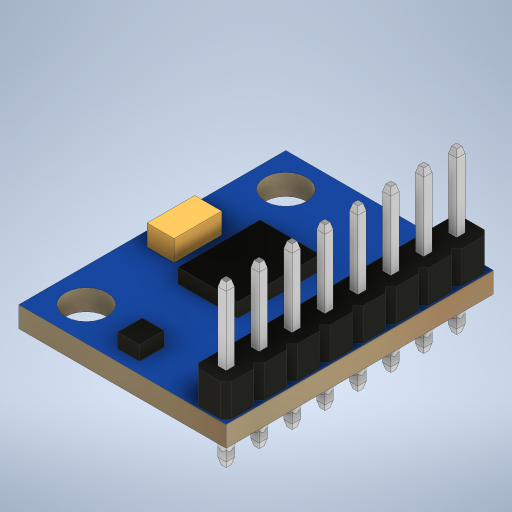
# Autodesk Inventor part: ACCELEROMETER
Saved by Autodesk Inventor 2023 (Build 270158000, 158)
## iProperties
Created: 2023-03-15
Part Number: ACCELEROMETER
Material: Generic
Document SubType Name: Modeling
Designer: Amos Yu
Density: 1 g/cm^3
Appearance: Default
Author: Amos Yu
Autodesk Inventor part; units mm, degrees
ref_plane "YZ Plane" through (0, 0, 0) normal (1, 0, 0) x (0, 1, 0)
ref_plane "XZ Plane" through (0, 0, 0) normal (0, 1, 0) x (-1, 0, 0)
ref_plane "XY Plane" through (0, 0, 0) normal (0, 0, 1) x (1, 0, 0)
sketch "Sketch1" plane through (0, 0, 0) normal (0, 1, 0) x (-1, 0, 0)
  line L0 (0, 0) -> (16, 0)
  line L1 (16, 0) -> (16, -20.6)
  line L2 (16, -20.6) -> (0, -20.6)
  line L3 (0, -20.6) -> (0, 0)
  circle A0 centre (13.4, -2.6) radius 1.6
  circle A1 centre (13.4, -18) radius 1.6
  point P0 (0, -10.3)
  dimension "d0" = 16
  dimension "d1" = 20.6
  dimension "d2" = 3.2
  dimension "d3" = 3.2
  dimension "d6" = 2.6
  dimension "d7" = 2.6
  dimension "d8" = 2.6
  constraints: 8 end point, 2 centre point, 2 parallel, 1 horizontal, 1 midpoint, 1 perpendicular, 1 vertical alignment
  measures "d0" distance of L1.end L2.end
  measures "d1" distance of L0.end L1.end
  measures "d2" diameter of A0
  measures "d3" diameter of A1
  measures "d6" distance from line of L0 A0.centre
  measures "d7" distance from line of L1 A0.centre
  measures "d8" distance from line of L2 A1.centre
extrude "Extrusion1" add sketch "Sketch1" along normal blind 1.6
sketch "Sketch2" plane through (0, 1.6, 0) normal (0, 1, 0) x (1, 0, 0)
  line L0 (-9.2513, 2.7827) -> (-7.5651, 2.7827)
  line L1 (-7.5651, 2.7827) -> (-7.5651, 0.8699)
  line L2 (-7.5651, 0.8699) -> (-9.2513, 0.8699)
  line L3 (-9.2513, 0.8699) -> (-9.2513, 2.7827)
  line L4 (-11.2621, 13.8736) -> (-6.6408, 13.8736)
  line L5 (-6.6408, 13.8736) -> (-6.6408, 7.5359)
  line L6 (-6.6408, 7.5359) -> (-11.2621, 7.5359)
  line L7 (-11.2621, 7.5359) -> (-11.2621, 13.8736)
  line L8 (-14.9036, 12.478) -> (-12.8178, 12.478)
  line L9 (-12.8178, 12.478) -> (-12.8178, 8.8062)
  line L10 (-12.8178, 8.8062) -> (-14.9036, 8.8062)
  line L11 (-14.9036, 8.8062) -> (-14.9036, 12.478)
  line L12 (-16, 20.6) -> (-16, 0) projected
  line L13 (-16, 0) -> (0, 0) projected
  point P0 (-8, 0)
  dimension "d11" = 1.6862
  dimension "d12" = 1.9128
  dimension "d13" = 6.3377
  dimension "d14" = 4.6212
  dimension "d15" = 2.0858
  dimension "d16" = 3.6718
  dimension "d17" = 1.0964
  dimension "d18" = 1.5558
  dimension "d19" = 7.5359
  dimension "d20" = 8.8062
  dimension "d21" = 0.8699
  dimension "d22" = 6.7487
  constraints: 24 end point, 6 parallel, 3 horizontal, 3 perpendicular, 1 midpoint
  measures "d11" distance of L1.end L2.end
  measures "d12" distance of L0.end L1.end
  measures "d13" distance of L4.end L5.end
  measures "d14" distance of L5.end L6.end
  measures "d15" distance of L9.end L10.end
  measures "d16" distance of L8.end L9.end
  measures "d17" distance between parallel lines of L12 L11
  measures "d18" distance between parallel lines of L9 L7
  measures "d19" distance between parallel lines of L13 L6
  measures "d20" distance between parallel lines of L13 L10
  measures "d21" distance from line of point (-8, 0) L2
  measures "d22" distance between parallel lines of L12 L3
extrude "Extrusion2" add sketch "Sketch2" along normal blind 1.1 contours L0 L1 L2 L3 | L4 L5 L6 L7
extrude "Extrusion3" add sketch "Sketch2" along normal blind 1.6 contours L8 L9 L10 L11
sketch "Sketch3" plane through (0, 1.6, 0) normal (0, 1, 0) x (1, 0, 0)
  line L0 (-2.2798, 0.14) -> (-0.5402, 0.14)
  line L1 (-0.5402, 0.14) -> (-0.14, 0.5402)
  line L2 (-0.14, 0.5402) -> (-0.14, 2.2798)
  line L3 (-0.14, 2.2798) -> (-0.5402, 2.68)
  line L4 (-0.5402, 2.68) -> (-2.2798, 2.68)
  line L5 (-2.2798, 2.68) -> (-2.68, 2.2798)
  line L6 (-2.68, 2.2798) -> (-2.68, 0.5402)
  line L7 (-2.68, 0.5402) -> (-2.2798, 0.14)
  line L8 (-16, 0) -> (0, 0) projected
  line L9 (0, 0) -> (0, 20.6) projected
  line L10 (-1.73, 1.09) -> (-1.09, 1.09)
  line L11 (-1.09, 1.09) -> (-1.09, 1.73)
  line L12 (-1.09, 1.73) -> (-1.73, 1.73)
  line L13 (-1.73, 1.73) -> (-1.73, 1.09)
  point P0 (-1.73, 1.41)
  point P1 (-2.68, 1.41)
  point P2 (-1.41, 1.73)
  point P3 (-1.41, 2.68)
  dimension "d31" = 135
  dimension "d32" = 0.566
  dimension "d33" = 2.54
  dimension "d34" = 2.54
  dimension "d35" = 0.566
  dimension "d36" = 0.566
  dimension "d37" = 0.566
  dimension "d38" = 0.14
  dimension "d39" = 0.14
  dimension "d42" = 0.64
  dimension "d43" = 0.64
  constraints: 24 end point, 5 perpendicular, 4 midpoint, 4 parallel, 2 horizontal, 1 horizontal alignment, 1 vertical alignment
  measures "d31" angle of L0 L7
  measures "d32" distance of L6.end L0.start
  measures "d33" distance between parallel lines of L4 L0
  measures "d34" distance between parallel lines of L6 L2
  measures "d35" distance of L4.end L5.end
  measures "d36" distance of L0.end L1.end
  measures "d37" distance of L2.end L3.end
  measures "d38" distance between parallel lines of L8 L0
  measures "d39" distance between parallel lines of L9 L2
  measures "d42" distance of L12.end L11.end
  measures "d43" distance of L11.end L10.end
extrude "Extrusion4" add sketch "Sketch3" along normal blind 2.5 contours L7 L6 L5 L4 L3 L2 L1 L0 | L13 L12 L11 L10
extrude "Extrusion5" add sketch "Sketch3" along normal blind 7.8 contours L13 L12 L11 L10
sketch "Sketch4" plane through (0, 9.4, 0) normal (0, 1, 0) x (1, 0, 0)
  line L0 (-1.73, 1.09) -> (-1.73, 1.73) projected
  line L1 (-1.09, 1.73) -> (-1.73, 1.73) projected
  line L2 (-1.73, 1.09) -> (-1.09, 1.09)
  line L3 (-1.09, 1.09) -> (-1.09, 1.73)
  line L4 (-1.09, 1.73) -> (-1.73, 1.73)
  line L5 (-1.73, 1.73) -> (-1.73, 1.09)
  point P0 (0, 0)
  constraints: 8 end point, 2 parallel, 1 horizontal, 1 perpendicular
extrude "Extrusion6" add sketch "Sketch4" along normal blind 0.5 draft -14
sketch "Sketch5" plane through (0, 0, 0) normal (0, -1, 0) x (1, 0, 0)
  circle A0 centre (-1.41, -1.41) radius 1
  line L0 (-0.14, -2.2798) -> (-0.14, -0.5402) projected
  line L1 (-0.5402, -0.14) -> (-2.2798, -0.14) projected
  point P0 (0, 0)
  point P1 (-0.14, -1.41)
  point P2 (-1.41, -0.14)
  dimension "d51" = 2
  constraints: 2 midpoint, 1 centre point, 1 horizontal alignment, 1 vertical alignment
  measures "d51" diameter of A0
extrude "Extrusion7" add sketch "Sketch3" against normal blind 3.6 contours L13 L12 L11 L10
sketch "Sketch6" plane through (0, -2, 0) normal (0, -1, 0) x (1, 0, 0)
  line L0 (-1.09, -1.09) -> (-1.73, -1.09) projected
  line L1 (-1.73, -1.09) -> (-1.73, -1.73) projected
  line L2 (-1.09, -1.09) -> (-1.73, -1.09)
  line L3 (-1.73, -1.09) -> (-1.73, -1.73)
  line L4 (-1.73, -1.73) -> (-1.09, -1.73)
  line L5 (-1.09, -1.73) -> (-1.09, -1.09)
  point P0 (0, 0)
  constraints: 8 end point, 2 parallel, 1 horizontal, 1 perpendicular
extrude "Extrusion8" add sketch "Sketch6" along normal blind 0.5 draft -14
extrude "Extrusion9" add sketch "Sketch5" along normal blind 2 draft -25
pattern_linear "Rectangular Pattern1" count 8 spacing 2.54 along (0, 0, -1) of "Extrusion4", "Extrusion5", "Extrusion6", "Extrusion9", "Extrusion8", "Extrusion7"
body "Solid1"
